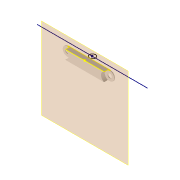
# Autodesk Inventor part: Cableholder_Ikealamp
Saved by Autodesk Inventor 2022 (Build 260153000, 153)
## iProperties
Created: 2022-12-21
Part Number: Cableholder_Ikealamp
Material: Generisch
Document SubType Name: Modeling
Designer: diederichbenedict
Density: 1 g/cm^3
Appearance: Vorgabe
Author: diederichbenedict
Autodesk Inventor part; units mm, degrees
ref_plane "YZ Plane" through (0, 0, 0) normal (1, 0, 0) x (0, 1, 0)
ref_plane "XZ Plane" through (0, 0, 0) normal (0, 1, 0) x (-1, 0, 0)
ref_plane "XY Plane" through (0, 0, 0) normal (0, 0, 1) x (1, 0, 0)
ref_plane "Arbeitsebene1" through (0, 0, 0) normal (0, 0, 1) x (1, 0, 0)
sketch "Skizze1" plane through (0, 0, 0) normal (0, 0, 1) x (1, 0, 0)
  circle A0 centre (17.5021, -9.9999) radius 1.45 projected
  circle A1 centre (-17.4978, -9.9998) radius 1.45 projected
  circle A2 centre (-17.4979, 10.0001) radius 1.45 projected
  circle A3 centre (17.5021, 10.0001) radius 1.45 projected
  arc A4 (-9.5, 21.063) -> (-12.4584, 22.8184) centre (-11.5, 21.063) ccw projected
  arc A5 (-12.4584, 22.8184) -> (12.4584, 22.8184) centre (0, 0) ccw projected
  arc A6 (12.4584, 22.8184) -> (9.5, 21.063) centre (11.5, 21.063) ccw projected
  line L0 (9.5, 21.063) -> (9.5, 17.6304) projected
  line L1 (9.5, 17.6304) -> (14, 17.6304) projected
  arc A7 (14, 10.6304) -> (14, 17.6304) centre (14, 14.1304) ccw projected
  line L2 (14, 10.6304) -> (9.5, 10.6304) projected
  line L3 (9.5, 10.6304) -> (9.5, -9) projected
  line L4 (9.5, -9) -> (-9.5, -9) projected
  line L5 (-9.5, -9) -> (-9.5, 10.6304) projected
  line L6 (-9.5, 10.6304) -> (-14, 10.6304) projected
  arc A8 (-14, 17.6304) -> (-14, 10.6304) centre (-14, 14.1304) ccw projected
  line L7 (-14, 17.6304) -> (-9.5, 17.6304) projected
  line L8 (-9.5, 17.6304) -> (-9.5, 21.063) projected
  circle A9 centre (-14, 14.1304) radius 1.4 projected
  circle A10 centre (14, 14.1304) radius 1.4 projected
  line L9 (-14, 14.1304) -> (14, 14.1304) construction
  line L10 (-14, 11.1304) -> (14, 11.1304)
  line L11 (14, 17.1304) -> (-14, 17.1304)
  arc A11 (-14, 17.1304) -> (-14, 11.1304) centre (-14, 14.1304) ccw
  arc A12 (14, 11.1304) -> (14, 17.1304) centre (14, 14.1304) ccw
  point P0 (0, 14.1304)
  dimension "d0" = 6
  constraints: 8 end point, 4 point on circle, 4 tangent, 2 centre point, 1 horizontal, 1 midpoint, 1 parallel
  measures "d0" diameter of A12
extrude "Extrusion1" add sketch "Skizze1" against normal blind 4 contours A11 L11 A12 L10
sketch "Skizze2" plane through (0, 0, 0) normal (0, 0, 1) x (1, 0, 0)
  arc A0 (14, 11.1304) -> (14, 17.1304) centre (14, 14.1304) ccw projected
  line L0 (14, 17.1304) -> (-14, 17.1304) projected
  arc A1 (-14, 17.1304) -> (-14, 11.1304) centre (-14, 14.1304) ccw projected
  line L1 (-14, 11.1304) -> (14, 11.1304) projected
  circle A2 centre (14, 14.1304) radius 1.4 projected
  circle A3 centre (-14, 14.1304) radius 1.4 projected
  point P0 (0, 0)
hole "Bohrung1" at (-14, 14.1304, 0) at (14, 14.1304, 0) direction (0, 0, -1) diameter 2.8 depth 7 tip angle 118 counterbore diameter 6.5 counterbore depth 2.5
sketch "Skizze3" plane through (-14, 17.1304, -4) normal (0, 1, 0) x (1, 0, 0)
  line L0 (1.25, -1.5) -> (1.25, -4) projected
  line L1 (26.75, -4) -> (1.25, -4) projected
  line L2 (26.75, -4) -> (26.75, -1.5) projected
  line L3 (26.75, -1.5) -> (28, -1.5) projected
  line L4 (28, -1.5) -> (28, 0) projected
  line L5 (0, 0) -> (28, 0) projected
  line L6 (0, -1.5) -> (0, 0) projected
  line L7 (0, -1.5) -> (1.25, -1.5) projected
  line L8 (-22.3971, 2) -> (50.3971, 2)
  circle A0 centre (14, 2) radius 2
  point P0 (14, -4)
  constraints: 2 end point, 1 centre point, 1 horizontal, 1 midpoint, 2 other
